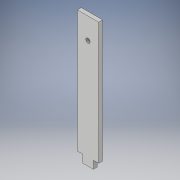
# Autodesk Inventor part: table_foot
Saved by Autodesk Inventor 2019.4 (Build 234330000, 330)
## iProperties
Created: 2019-12-14
Part Number: table_foot
Material: Generic
Document SubType Name: Modeling
Designer: fabfarm
Density: 1 g/cm^3
Appearance: Default
Author: fabfarm
Autodesk Inventor part; units mm, degrees
ref_plane "YZ Plane" through (0, 0, 0) normal (1, 0, 0) x (0, 1, 0)
ref_plane "XZ Plane" through (0, 0, 0) normal (0, 1, 0) x (-1, 0, 0)
ref_plane "XY Plane" through (0, 0, 0) normal (0, 0, 1) x (1, 0, 0)
sketch "Sketch1" plane through (0, 0, 0) normal (0, 0, 1) x (1, 0, 0)
  line L0 (0, 0) -> (0, 575)
  line L1 (0, 575) -> (100, 575)
  line L2 (100, 575) -> (100, 0)
  line L3 (100, 0) -> (0, 0)
  dimension "d0" = 575
  dimension "d1" = 100
  constraints: 8 end point, 3 perpendicular, 1 vertical
  measures "d0" distance of L1.end L2.end
  measures "d1" distance of L2.end L0.start
extrude "Extrusion1" add sketch "Sketch1" along normal blind 18.55
sketch "Sketch2" plane through (0, 0, 18.55) normal (0, 0, 1) x (1, 0, 0)
  circle A0 centre (50, 475) radius 10
  line L0 (0, 575) -> (0, 0) projected
  line L1 (0, 475) -> (100, 475) construction
  line L2 (100, 0) -> (100, 575) projected
  line L3 (100, 575) -> (0, 575) projected
  dimension "d4" = 50
  dimension "d5" = 100
  dimension "d6" = 20
  constraints: 2 end point, 2 point on line, 1 centre point, 1 horizontal, 1 midpoint
  measures "d4" distance from line of L0 A0.centre
  measures "d5" distance between parallel lines of L3 L1
  measures "d6" diameter of A0
extrude "Extrusion2" cut sketch "Sketch2" against normal blind 100
sketch "Sketch3" plane through (0, 0, 18.55) normal (0, 0, 1) x (1, 0, 0)
  line L0 (0, 0) -> (100, 0) projected
  line L1 (25, 0) -> (75, 0)
  line L2 (75, 0) -> (75, -37.1)
  line L3 (75, -37.1) -> (25, -37.1)
  line L4 (25, -37.1) -> (25, 0)
  line L5 (0, 575) -> (0, 0) projected
  line L6 (100, 0) -> (100, 575) projected
  dimension "d9" = 25
  dimension "d10" = 25
  dimension "d11" = 37.1
  constraints: 8 end point, 2 parallel, 1 horizontal, 1 perpendicular, 1 point on line
  measures "d9" distance between parallel lines of L5 L4
  measures "d10" distance between parallel lines of L2 L6
  measures "d11" distance of L1.end L2.end
extrude "Extrusion3" add sketch "Sketch3" against normal blind 18.55
body "Solid1"
